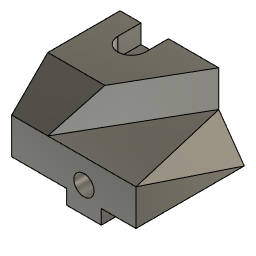
NCV-14 v1 (Autodesk Fusion 360 design; units mm, degrees)
Autodesk Fusion 360 part; units mm, degrees
sketch "Sketch1" plane through (0, 0, 0) normal (0, 0, 1) x (1, 0, 0)
  line L0 (0, 0) -> (86, 0)
  line L1 (86, 0) -> (86, -75)
  line L2 (86, -75) -> (0, -75)
  line L3 (0, -75) -> (0, 0)
  line L4 (68.3013, 0) -> (25, -75)
  line L5 (14.5, 0) -> (14.5, -16)
  line L6 (33.5, 0) -> (33.5, -16)
  arc A0 (14.5, -16) -> (33.5, -16) centre (24, -16) ccw
  line L7 (38, 0) -> (62, 0)
  line L8 (62, 0) -> (62, -75)
  line L9 (62, -75) -> (38, -75)
  line L10 (38, -75) -> (38, 0)
  line L11 (86, -75) -> (68.3013, 0)
  dimension "d1" = 75
  dimension "d2" = 86
  dimension "d3" = 60
  dimension "d4" = 25
  dimension "d5" = 19
  dimension "d6" = 16
  dimension "d7" = 24
  dimension "d8" = 38
  dimension "d9" = 62
  dimension "d22" = 68.3013
  constraint horizontal L0
  constraint vertical L1
  constraint horizontal L2
  constraint vertical L3
  constraint coincident L0.start L3.end
  constraint coincident L0 L4.start
  constraint coincident L2 L4.end
  constraint coincident L0 L5.start
  constraint coincident L0 L6.start
  constraint vertical L6
  constraint vertical L5
  constraint tangent L5 A0
  constraint tangent L6 A0
  constraint horizontal L7
  constraint vertical L8
  constraint horizontal L9
  constraint vertical L10
  constraint coincident L2 L8.end
  constraint coincident L0 L7.start
  measures "d1" distance of L0.start L2.end
  measures "d2" distance of L0.start L0.end
  measures "d3" angle of L2 L4
  measures "d4" horizontal distance of L0.start L4.end
  measures "d5" diameter of A0
  measures "d6" vertical distance of L0.start A0.centre
  measures "d7" horizontal distance of L0.start A0.centre
  measures "d8" distance of L0.start L7.start
  measures "d9" distance of L0.start L7.end
  measures "d22" distance of L0.start L4.start
sketch "Sketch2" plane through (0, 0, 0) normal (0, 1, 0) x (1, 0, 0)
  circle A0 centre (50, 17) radius 7
  line L0 (86, 0) -> (86, 25)
  line L1 (86, 25) -> (68.3013, 0)
  line L2 (68.3013, 0) -> (86, 0)
  dimension "d18" = 14
  dimension "d19" = 50
  dimension "d20" = 17
  dimension "d21" = 86
  dimension "d23" = 68.3013
  dimension "d24" = 25
  dimension "d25" = 25
  constraint vertical L0
  constraint horizontal L2
  measures "d18" diameter of A0
  measures "d19" horizontal distance of A0.centre origin
  measures "d20" vertical distance of A0.centre origin
  measures "d21" distance of origin L0.start
  measures "d23" distance of origin L1.end
  measures "d24" vertical distance of origin L0.end
  measures "d25" distance of L0.start L0.end
extrude "Extrude1" add sketch "Sketch1" along normal blind 25 contours L0 L2 L3 L4 L5 L6 A0 L10 | L0 L4 L7 L8 L10 | L0 L4 L8 makes body 1
extrude "Extrude2" add sketch "Sketch1" along normal blind 12 contours L0 L5 L6 A0 bodies 1
extrude "Extrude3" add sketch "Sketch1" against normal blind 25 separate body contours L0 L2 L3 L4 L5 L6 A0 L10 | L0 L5 L6 A0 | L2 L4 L10 | L0 L4 L8 | L2 L4 L8 L11 | L0 L1 L11 makes body 2 at (12.6667, -25, 0) makes body 3 at (62, -25, -8.3333)
extrude "Extrude4" add sketch "Sketch1" against normal blind 35 contours L0 L4 L7 L8 L10 | L2 L4 L8 L9 L10 bodies 1 3 2
extrude "Extrude5" cut sketch "Sketch2" against normal through all contours A0 bodies 1
loft "Loft1" cut profiles "Sketch1", "Sketch2" section 1 contours L0 L1 L11 section 2 contours L0 L1 L2 bodies 1
chamfer "Chamfer1" distance 25 angle 45 1 edges at (12.5, -75, 25) on bodies 1
equation "d2 = 38 mm + 24 mm + 24 mm"
equation "d5 = ( 9.5 * 2 ) * 1 mm"
equation "d9 = 38 mm + 24 mm"
equation "d12 = 25 mm - 13 mm"
equation "d16 = -25 mm - 10 mm"
equation "d19 = 12 mm + 38 mm"
equation "d20 = 10 mm + 25 mm - 18 mm"
equation "d21 = 38 mm + 24 mm + 24 mm"
equation "d23 = d22"
